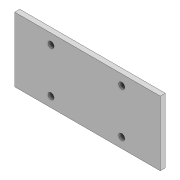
# Autodesk Inventor part: second
Saved by Autodesk Inventor 2020 (Build 240168000, 168)
## iProperties
Created: 2021-12-09
Part Number: second
Material: Generic
Document SubType Name: Modeling
Designer: NIKHIL VINOD
Density: 1 g/cm^3
Appearance: Default
Author: NIKHIL VINOD
Autodesk Inventor part; units mm, degrees
ref_plane "YZ Plane" through (0, 0, 0) normal (1, 0, 0) x (0, 1, 0)
ref_plane "XZ Plane" through (0, 0, 0) normal (0, 1, 0) x (-1, 0, 0)
ref_plane "XY Plane" through (0, 0, 0) normal (0, 0, 1) x (1, 0, 0)
sketch "Sketch1" plane through (0, 0, 0) normal (0, 0, 1) x (1, 0, 0)
  line L0 (0, 0) -> (-144, 0)
  line L1 (-144, 0) -> (-144, 64)
  line L2 (-144, 64) -> (0, 64)
  line L3 (0, 64) -> (0, 0)
  circle A0 centre (-108, 54) radius 3
  circle A1 centre (-38, 54) radius 3
  circle A2 centre (-108, 10) radius 3
  circle A3 centre (-38, 10) radius 3
  dimension "d0" = 144
  dimension "d1" = 64
  dimension "d2" = 6
  dimension "d3" = 36
  dimension "d4" = 10
  dimension "d7" = 70
  dimension "d10" = 44
  constraints: 8 end point, 4 centre point, 2 horizontal, 2 parallel, 1 perpendicular, 1 vertical, 6 other
  measures "d0" distance of L1.end L2.end
  measures "d1" distance of L0.end L1.end
  measures "d2" diameter of A0
  measures "d3" distance from line of L1 A0.centre
  measures "d4" distance from line of L2 A0.centre
  measures "d7" distance of A0.centre A1.centre
  measures "d10" distance of A0.centre A2.centre
extrude "Extrusion1" add sketch "Sketch1" along normal blind 5
body "Solid1"
